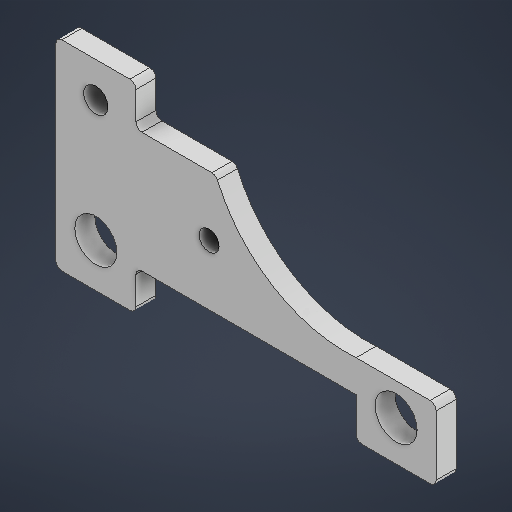
# Autodesk Inventor part: lateralCanhao
Saved by Autodesk Inventor 2026.2 (Build 302298000, 298)
## iProperties
Created: 2026-09-04
Part Number: lateralCanhao
Material: Genérico
Document SubType Name: Modeling
Designer: IFSP
Density: 1 g/cm^3
Appearance: Padrão
Author: IFSP
Autodesk Inventor part; units mm, degrees
ref_plane "YZ Plane" through (0, 0, 0) normal (1, 0, 0) x (0, 1, 0)
ref_plane "XZ Plane" through (0, 0, 0) normal (0, 1, 0) x (-1, 0, 0)
ref_plane "XY Plane" through (0, 0, 0) normal (0, 0, 1) x (1, 0, 0)
sketch "Esboço1" plane through (0, 0, 0) normal (0, 1, 0) x (-1, 0, 0)
  point P0 (0, 0)
sketch "Esboço2" plane through (0, 0, 0) normal (0, 0, 1) x (1, 0, 0)
  line L0 (0, 0) -> (20, 0)
  line L1 (20, 0) -> (20, 10)
  line L2 (20, 10) -> (75, 10)
  line L3 (75, 10) -> (75, 0)
  line L4 (75, 0) -> (95, 0)
  line L5 (95, 0) -> (95, 18)
  line L6 (95, 18) -> (75, 18)
  line L7 (0, 0) -> (0, 50)
  line L8 (0, 50) -> (20, 50)
  line L9 (20, 50) -> (20, 40)
  line L10 (20, 40) -> (40, 40)
  arc A0 (40, 40) -> (75, 18) centre (72.5309, 52.9128) ccw
  circle A1 centre (10, 41.2323) radius 3.05
  circle A2 centre (10, 10.8785) radius 5.25
  circle A3 centre (85, 10) radius 5.25
  circle A4 centre (38.286, 25) radius 2.5
  dimension "d0" = 20
  dimension "d1" = 10
  dimension "d2" = 55
  dimension "d3" = 10
  dimension "d4" = 20
  dimension "d5" = 18
  dimension "d6" = 20
  dimension "d7" = 50
  dimension "d8" = 20
  dimension "d9" = 10
  dimension "d10" = 20
  dimension "d11" = 35
  dimension "d12" = 6.1
  dimension "d13" = 10.5
  dimension "d14" = 10.5
  dimension "d15" = 5
  constraints: 22 end point, 6 perpendicular, 5 centre point, 3 point on line, 2 point on circle, 1 horizontal, 1 vertical
  measures "d0" distance of L0.start L0.end
  measures "d1" distance of L0.end L1.end
  measures "d2" distance of L1.end L2.end
  measures "d3" distance of L2.end L3.end
  measures "d4" distance of L3.end L4.end
  measures "d5" distance of L4.end L5.end
  measures "d6" distance of L5.end L6.end
  measures "d7" distance of L0.start L7.end
  measures "d8" distance of L7.end L8.end
  measures "d9" distance of L8.end L9.end
  measures "d10" distance of L9.end L10.end
  measures "d11" radius of A0
  measures "d12" diameter of A1
  measures "d13" diameter of A2
  measures "d14" diameter of A3
  measures "d15" diameter of A4
extrude "Extrusão1" add sketch "Esboço2" along normal blind 5
fillet "Arredondamento1" radius 1.5 2 edges at (0, 50, 2.5) (20, 50, 2.5)
fillet "Arredondamento2" radius 1.5 8 edges at (20, 40, 2.5) (40, 40, 2.5) (95, 0, 2.5) (75, 0, 2.5) (20, 0, 2.5) (20, 10, 2.5) (95, 18, 2.5) (0, 0, 2.5)
